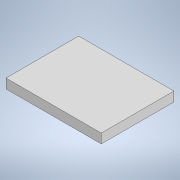
# Autodesk Inventor part: RoadBot Pneumatic Module - Connection Bay Cover- r1
Saved by Autodesk Inventor 2020 (Build 240168000, 168)
## iProperties
Created: 2022-04-02
Part Number: RoadBot Pneumatic Module - Connection Bay Cover- r1
Material: Generic
Document SubType Name: Modeling
Designer: Beaucage
Density: 1 g/cm^3
Appearance: Default
Author: Beaucage
Autodesk Inventor part; units mm, degrees
ref_plane "YZ Plane" through (0, 0, 0) normal (1, 0, 0) x (0, 1, 0)
ref_plane "XZ Plane" through (0, 0, 0) normal (0, 1, 0) x (-1, 0, 0)
ref_plane "XY Plane" through (0, 0, 0) normal (0, 0, 1) x (1, 0, 0)
sketch "Sketch1" plane through (0, 0, 0) normal (0, 1, 0) x (-1, 0, 0)
  line L0 (0, 0) -> (31.9786, 0)
  line L1 (31.9786, 0) -> (31.9786, -24.4094)
  line L2 (31.9786, -24.4094) -> (0, -24.4094)
  line L3 (0, -24.4094) -> (0, 0)
  dimension "d0" = 31.9786
  dimension "d1" = 24.4094
  constraints: 8 end point, 2 parallel, 1 horizontal, 1 perpendicular
  measures "d0" distance of L1.end L2.end
  measures "d1" distance of L0.end L1.end
extrude "Extrusion1" add sketch "Sketch1" along normal blind 3.175
body "Solid1"
